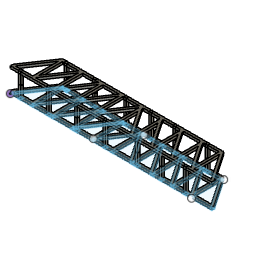
yamato (Autodesk Fusion 360 design; units mm, degrees)
Autodesk Fusion 360 part; units mm, degrees
note: some values were not read from the file. Chosen so that the rebuilt part matches the saved one: which bodies a step acts on; a direction.
sketch "Sketch1" plane through (0, 0, 0) normal (0, 0, 1) x (1, 0, 0)
  line L0 (0, 0) -> (250, 0)
  line L1 (250, 0) -> (250, 3)
  line L2 (250, 3) -> (0, 3)
  line L3 (0, 3) -> (0, 0)
  line L4 (25, 40) -> (225, 40)
  line L5 (225, 40) -> (225, 37)
  line L6 (225, 37) -> (25, 37)
  line L7 (25, 37) -> (25, 40)
  line L8 (225, 40) -> (250, 3)
  line L9 (250, 3) -> (247.5142, 1.3204)
  line L10 (247.5142, 1.3204) -> (222.5142, 38.3204)
  line L11 (222.5142, 38.3204) -> (225, 40)
  line L12 (25, 40) -> (0, 3)
  line L13 (0, 3) -> (2.4858, 1.3204)
  line L14 (2.4858, 1.3204) -> (27.4858, 38.3204)
  line L15 (27.4858, 38.3204) -> (25, 40)
  line L16 (50, 40) -> (53, 40)
  line L17 (53, 40) -> (53, 0)
  line L18 (53, 0) -> (50, 0)
  line L19 (50, 0) -> (50, 40)
  line L20 (75, 0) -> (75, 40)
  line L21 (78, 40) -> (78, 0)
  line L22 (75, 40) -> (78, 40)
  line L23 (78, 0) -> (75, 0)
  line L24 (100, 40) -> (103, 40)
  line L25 (100, 0) -> (100, 40)
  line L26 (103, 40) -> (103, 0)
  line L27 (103, 0) -> (100, 0)
  line L28 (128, 0) -> (125, 0)
  line L29 (125, 0) -> (125, 40)
  line L30 (128, 40) -> (128, 0)
  line L31 (125, 40) -> (128, 40)
  line L32 (150, 40) -> (153, 40)
  line L33 (150, 0) -> (150, 40)
  line L34 (153, 40) -> (153, 0)
  line L35 (153, 0) -> (150, 0)
  line L36 (178, 0) -> (175, 0)
  line L37 (175, 0) -> (175, 40)
  line L38 (178, 40) -> (178, 0)
  line L39 (175, 40) -> (178, 40)
  line L40 (200, 40) -> (203, 40)
  line L41 (200, 0) -> (200, 40)
  line L42 (203, 40) -> (203, 0)
  line L43 (203, 0) -> (200, 0)
  line L44 (225, 0) -> (225, 40)
  line L45 (25, 40) -> (28, 40)
  line L46 (25, 0) -> (25, 40)
  line L47 (28, 40) -> (28, 0)
  line L48 (28, 0) -> (25, 0)
  line L49 (222, 40) -> (225, 40)
  line L50 (222, 0) -> (222, 40)
  line L51 (225, 0) -> (222, 0)
  line L52 (197.5142, 38.3204) -> (200, 40)
  line L53 (200, 40) -> (225, 3)
  line L54 (222.5142, 1.3204) -> (197.5142, 38.3204)
  line L55 (225, 3) -> (222.5142, 1.3204)
  line L56 (172.5142, 38.3204) -> (175, 40)
  line L57 (175, 40) -> (200, 3)
  line L58 (197.5142, 1.3204) -> (172.5142, 38.3204)
  line L59 (200, 3) -> (197.5142, 1.3204)
  line L60 (147.5142, 38.3204) -> (150, 40)
  line L61 (150, 40) -> (175, 3)
  line L62 (172.5142, 1.3204) -> (147.5142, 38.3204)
  line L63 (175, 3) -> (172.5142, 1.3204)
  line L64 (122.5142, 38.3204) -> (125, 40)
  line L65 (125, 40) -> (150, 3)
  line L66 (147.5142, 1.3204) -> (122.5142, 38.3204)
  line L67 (150, 3) -> (147.5142, 1.3204)
  line L68 (25, 3) -> (27.4858, 1.3204)
  line L69 (27.4858, 1.3204) -> (52.4858, 38.3204)
  line L70 (50, 40) -> (25, 3)
  line L71 (52.4858, 38.3204) -> (50, 40)
  line L72 (50, 3) -> (52.4858, 1.3204)
  line L73 (52.4858, 1.3204) -> (77.4858, 38.3204)
  line L74 (75, 40) -> (50, 3)
  line L75 (77.4858, 38.3204) -> (75, 40)
  line L76 (75, 3) -> (77.4858, 1.3204)
  line L77 (77.4858, 1.3204) -> (102.4858, 38.3204)
  line L78 (100, 40) -> (75, 3)
  line L79 (102.4858, 38.3204) -> (100, 40)
  line L80 (0, 3) -> (2.4858, 1.3204)
  line L81 (2.4858, 1.3204) -> (27.4858, 38.3204)
  line L82 (25, 40) -> (0, 3)
  line L83 (27.4858, 38.3204) -> (25, 40)
  line L84 (100, 40) -> (75, 3)
  line L85 (75, 3) -> (77.4858, 1.3204)
  line L86 (77.4858, 1.3204) -> (102.4858, 38.3204)
  line L87 (102.4858, 38.3204) -> (100, 40)
  line L88 (127.4858, 38.3204) -> (125, 40)
  line L89 (125, 40) -> (100, 3)
  line L90 (102.4858, 1.3204) -> (127.4858, 38.3204)
  line L91 (100, 3) -> (102.4858, 1.3204)
  line L92 (30, 40) -> (33, 40)
  line L93 (33, 40) -> (33, 37)
  line L94 (33, 37) -> (30, 37)
  line L95 (30, 37) -> (30, 40)
  line L96 (65, 37) -> (65, 40)
  line L97 (65, 40) -> (68, 40)
  line L98 (68, 40) -> (68, 37)
  line L99 (68, 37) -> (65, 37)
  line L100 (30, 37) -> (30, 40)
  line L101 (30, 40) -> (33, 40)
  line L102 (33, 40) -> (33, 37)
  line L103 (33, 37) -> (30, 37)
  line L104 (104, 37) -> (104, 40)
  line L105 (104, 40) -> (107, 40)
  line L106 (107, 40) -> (107, 37)
  line L107 (107, 37) -> (104, 37)
  line L108 (135, 37) -> (135, 40)
  line L109 (135, 40) -> (138, 40)
  line L110 (138, 40) -> (138, 37)
  line L111 (138, 37) -> (135, 37)
  line L112 (165, 37) -> (165, 40)
  line L113 (165, 40) -> (168, 40)
  line L114 (168, 40) -> (168, 37)
  line L115 (168, 37) -> (165, 37)
  line L116 (205, 37) -> (205, 40)
  line L117 (205, 40) -> (208, 40)
  line L118 (208, 40) -> (208, 37)
  line L119 (208, 37) -> (205, 37)
  line L120 (30, 37) -> (30, 40)
  line L121 (30, 40) -> (33, 40)
  line L122 (33, 40) -> (33, 37)
  line L123 (33, 37) -> (30, 37)
  line L124 (10, 0) -> (10, 3)
  line L125 (10, 3) -> (13, 3)
  line L126 (13, 3) -> (13, 0)
  line L127 (13, 0) -> (10, 0)
  line L128 (45, 0) -> (45, 3)
  line L129 (45, 3) -> (48, 3)
  line L130 (48, 3) -> (48, 0)
  line L131 (48, 0) -> (45, 0)
  line L132 (80, 0) -> (80, 3)
  line L133 (80, 3) -> (83, 3)
  line L134 (83, 3) -> (83, 0)
  line L135 (83, 0) -> (80, 0)
  line L136 (115, 0) -> (115, 3)
  line L137 (115, 3) -> (118, 3)
  line L138 (118, 3) -> (118, 0)
  line L139 (118, 0) -> (115, 0)
  line L140 (155, 0) -> (155, 3)
  line L141 (155, 3) -> (158, 3)
  line L142 (158, 3) -> (158, 0)
  line L143 (158, 0) -> (155, 0)
  line L144 (185, 0) -> (185, 3)
  line L145 (185, 3) -> (188, 3)
  line L146 (188, 3) -> (188, 0)
  line L147 (188, 0) -> (185, 0)
  line L148 (215, 0) -> (215, 3)
  line L149 (215, 3) -> (218, 3)
  line L150 (218, 3) -> (218, 0)
  line L151 (218, 0) -> (215, 0)
  line L152 (30, 37) -> (30, 40)
  line L153 (30, 40) -> (33, 40)
  line L154 (33, 40) -> (33, 37)
  line L155 (33, 37) -> (30, 37)
  dimension "d1" = 250
  dimension "d2" = 3
  dimension "d3" = 200
  dimension "d4" = 3
  dimension "d5" = 3
  dimension "d7" = 3
  dimension "d8" = 3
  dimension "d9" = 3
  dimension "d10" = 3
  dimension "d11" = 3
  dimension "d12" = 3
  dimension "d13" = 3
  dimension "d14" = 3
  dimension "d16" = 3
  dimension "d17" = 3
  dimension "d18" = 3
  dimension "d19" = 3
  dimension "d20" = 3
  dimension "d21" = 3
  dimension "d22" = 3
  dimension "d23" = 3
  dimension "d24" = 3
  dimension "d25" = 3
  dimension "d26" = 3
  dimension "d27" = 3
  dimension "d32" = 3
  dimension "d33" = 3
  dimension "d34" = 3
  dimension "d35" = 3
  dimension "d36" = 3
  dimension "d37" = 3
  dimension "d38" = 3
  dimension "d39" = 3
  dimension "d40" = 3
  dimension "d41" = 3
  dimension "d42" = 3
  dimension "d43" = 3
  dimension "d44" = 3
  dimension "d45" = 3
  dimension "d46" = 3
  dimension "d47" = 3
  constraint coincident L0.start L3.end
  constraint perpendicular L8 L9
  constraint parallel L8 L10
  constraint parallel L9 L11
  constraint perpendicular L12 L13
  constraint parallel L12 L14
  constraint parallel L13 L15
  constraint perpendicular L16 L17
  constraint parallel L16 L18
  constraint parallel L17 L19
  constraint parallel L4 L16
  constraint coincident L4 L16.start
  constraint perpendicular L21 L22
  constraint parallel L22 L23
  constraint parallel L20 L21
  constraint perpendicular L24 L26
  constraint parallel L24 L27
  constraint parallel L25 L26
  constraint perpendicular L30 L31
  constraint parallel L28 L31
  constraint parallel L29 L30
  constraint perpendicular L32 L34
  constraint parallel L32 L35
  constraint parallel L33 L34
  constraint perpendicular L38 L39
  constraint parallel L36 L39
  constraint parallel L37 L38
  constraint perpendicular L40 L42
  constraint parallel L40 L43
  constraint parallel L41 L42
  constraint perpendicular L45 L47
  constraint parallel L45 L48
  constraint parallel L46 L47
  constraint parallel L49 L51
  constraint perpendicular L53 L55
  constraint parallel L53 L54
  constraint parallel L52 L55
  constraint perpendicular L57 L59
  constraint parallel L57 L58
  constraint parallel L56 L59
  constraint perpendicular L61 L63
  constraint parallel L61 L62
  constraint parallel L60 L63
  constraint perpendicular L65 L67
  constraint parallel L65 L66
  constraint parallel L64 L67
  constraint perpendicular L68 L70
  constraint parallel L69 L70
  constraint parallel L68 L71
  constraint perpendicular L72 L74
  constraint parallel L73 L74
  constraint parallel L72 L75
  constraint perpendicular L76 L78
  constraint parallel L77 L78
  constraint parallel L76 L79
  constraint perpendicular L80 L82
  constraint parallel L81 L82
  constraint parallel L80 L83
  constraint perpendicular L84 L85
  constraint parallel L84 L86
  constraint parallel L85 L87
  constraint horizontal L92
  constraint vertical L93
  constraint horizontal L94
  constraint vertical L95
  constraint coincident L4 L92.start
  constraint horizontal L97
  constraint vertical L98
  constraint horizontal L99
  constraint vertical L96
  constraint horizontal L101
  constraint vertical L102
  constraint horizontal L103
  constraint vertical L100
  constraint horizontal L105
  constraint vertical L106
  constraint horizontal L107
  constraint vertical L104
  constraint horizontal L109
  constraint vertical L110
  constraint horizontal L111
  constraint vertical L108
  constraint horizontal L113
  constraint vertical L114
  constraint horizontal L115
  constraint vertical L112
  constraint horizontal L117
  constraint vertical L118
  constraint horizontal L119
  constraint vertical L116
  constraint horizontal L121
  constraint vertical L122
  constraint horizontal L123
  constraint vertical L120
  constraint horizontal L125
  constraint vertical L126
  constraint horizontal L127
  constraint vertical L124
  constraint horizontal L129
  constraint vertical L130
  constraint horizontal L131
  constraint vertical L128
  constraint horizontal L133
  constraint vertical L134
  constraint horizontal L135
  constraint vertical L132
  constraint horizontal L137
  constraint vertical L138
  constraint horizontal L139
  constraint vertical L136
  constraint horizontal L141
  constraint vertical L142
  constraint horizontal L143
  constraint vertical L140
  constraint horizontal L145
  constraint vertical L146
  constraint horizontal L147
  constraint vertical L144
  constraint horizontal L149
  constraint vertical L150
  constraint horizontal L151
  constraint vertical L148
  constraint horizontal L153
  constraint vertical L154
  constraint horizontal L155
  constraint vertical L152
  measures "d1" distance of L0.start L0.end
  measures "d2" distance of L0.start L2.end
  measures "d3" distance of L4.start L4.end
  measures "d4" distance of L4.start L6.end
  measures "d5" distance of L4.end L10.end
  measures "d7" distance of L4.start L14.end
  measures "d8" distance of L16.start L16.end
  measures "d9" distance of L21.start L20.end
  measures "d10" distance of L24.end L24.start
  measures "d11" distance of L29.end L30.start
  measures "d12" distance of L32.end L32.start
  measures "d13" distance of L37.end L38.start
  measures "d14" distance of L40.end L40.start
  measures "d16" distance of L45.end L4.start
  measures "d17" distance of L49.start L4.end
  measures "d18" distance of L52.start L40.start
  measures "d19" distance of L56.start L37.end
  measures "d20" distance of L60.start L32.start
  measures "d21" distance of L64.start L29.end
  measures "d22" distance of L16.start L69.end
  measures "d23" distance of L20.end L73.end
  measures "d24" distance of L24.start L77.end
  measures "d25" distance of L4.start L14.end
  measures "d26" distance of L24.start L77.end
  measures "d27" distance of L29.end L88.start
  measures "d32" distance of L92.start L92.end
  measures "d33" distance of L96.end L97.end
  measures "d34" distance of L92.start L92.end
  measures "d35" distance of L104.end L105.end
  measures "d36" distance of L108.end L109.end
  measures "d37" distance of L112.end L113.end
  measures "d38" distance of L116.end L117.end
  measures "d39" distance of L92.start L92.end
  measures "d40" distance of L124.end L125.end
  measures "d41" distance of L128.end L129.end
  measures "d42" distance of L132.end L133.end
  measures "d43" distance of L136.end L137.end
  measures "d44" distance of L140.end L141.end
  measures "d45" distance of L144.end L145.end
  measures "d46" distance of L148.end L149.end
  measures "d47" distance of L92.start L92.end
extrude "Extrude2" add sketch "Sketch1" along normal blind 15 contours L0 L2 L124 L125 L126 L127 | L4 L6 L92 L93 L94 L95 L100 L101 L102 L103 L120 L121 L122 L123 L152 L153 L154 L155 | L0 L2 L128 L129 L130 L131 | L4 L6 L96 L97 L98 L99 | L0 L2 L132 L133 L134 L135 | L4 L6 L104 L105 L106 L107 | L0 L2 L136 L137 L138 L139 | L4 L6 L108 L109 L110 L111 | L0 L2 L140 L141 L142 L143 | L4 L6 L112 L113 L114 L115 | L4 L6 L116 L117 L118 L119 | L0 L2 L148 L149 L150 L151 makes body 1 at (166, 40, 5) makes body 2 at (117, 3, 5) makes body 3 at (66, 40, 5) makes body 4 at (12, 3, 5) makes body 5 at (106, 37, 5) makes body 6 at (206, 40, 5) makes body 7 at (157, 3, 5) makes body 8 at (82, 3, 5) makes body 9 at (31, 40, 5) makes body 10 at (47, 3, 5) makes body 11 at (136, 40, 5) makes body 12 at (217, 3, 5)
extrude "Extrude1" add sketch "Sketch1" along normal blind 3 separate body contours L0 L2 L3 L13 L14 L80 L81 L124 | L0 L2 L124 L125 L126 L127 | L2 L7 L12 L14 L46 L81 L82 | L2 L13 L14 L80 L81 | L0 L2 L46 L126 | L6 L7 L14 L15 L46 L81 L83 | L4 L6 L14 L15 L45 L47 L81 L83 | L0 L46 L47 L48 L68 L69 | L6 L14 L46 L81 | L6 L14 L46 L47 L70 L81 | L4 L6 L47 L95 L100 L120 L152 | L0 L2 L47 L69 L128 | L2 L47 L70 | L2 L47 L68 L69 | L4 L6 L92 L93 L94 L95 L100 L101 L102 L103 L120 L121 L122 L123 L152 L153 L154 L155 | L0 L2 L128 L129 L130 L131 | L2 L47 L69 | L2 L6 L19 L47 L69 L70 | L4 L6 L70 L93 L102 L122 L154 | L0 L2 L19 L130 | L6 L19 L70 | L6 L19 L69 L71 | L4 L6 L16 L17 L69 L71 | L0 L17 L18 L19 L72 L73 | L6 L17 L19 L69 L74 | L6 L19 L69 | L4 L6 L17 L96 | L0 L2 L17 L20 L73 | L2 L17 L74 | L2 L17 L72 L73 | L4 L6 L96 L97 L98 L99 | L0 L20 L21 L23 L76 L77 L85 L86 | L2 L17 L73 | L2 L6 L17 L20 L73 L74 | L4 L6 L74 L98 | L0 L2 L21 L77 L86 L132 | L2 L21 L78 L84 | L2 L21 L76 L77 L85 L86 | L6 L20 L21 L73 L78 L84 | L6 L20 L74 | L6 L20 L73 L75 | L4 L6 L21 L22 L73 L75 | L0 L2 L132 L133 L134 L135 | L2 L21 L77 L86 | L2 L6 L21 L25 L77 L78 L84 L86 | L6 L20 L73 | L4 L6 L21 L78 L84 | L0 L2 L25 L134 | L6 L25 L78 L84 | L6 L25 L77 L79 L86 L87 | L4 L6 L24 L26 L77 L79 L86 L87 | L0 L25 L26 L27 L90 L91 | L6 L25 L26 L77 L86 L89 | L6 L25 L77 L86 | L4 L6 L26 L104 | L0 L2 L26 L90 L136 | L2 L26 L89 | L2 L26 L90 L91 | L4 L6 L104 L105 L106 L107 | L0 L2 L136 L137 L138 L139 | L2 L26 L90 | L2 L6 L26 L66 L89 L90 | L4 L6 L64 L66 L89 L106 | L0 L2 L29 L138 | L6 L66 L89 | L6 L29 L65 L90 | L64 L66 L89 | L65 L88 L90 | L4 L6 L30 L31 L65 L88 L90 | L6 L29 L66 L89 | L0 L2 L28 L29 L30 | L2 L29 L30 L66 | L6 L29 L66 | L6 L30 L65 L66 L90 | L6 L29 L90 | L4 L6 L30 L108 | L6 L65 L90 | L0 L2 L30 L33 L66 L67 | L2 L30 L65 L66 | L4 L6 L108 L109 L110 L111 | L6 L30 L65 | L0 L2 L33 L34 L35 | L2 L66 L67 | L4 L6 L60 L62 L110 | L0 L2 L34 L140 | L2 L33 L34 L62 | L6 L33 L61 | L6 L33 L60 L62 | L4 L6 L32 L34 L61 | L0 L2 L140 L141 L142 L143 | L6 L33 L62 | L6 L33 L34 L61 L62 | L4 L6 L34 L112 | L6 L34 L61 | L0 L2 L37 L62 L63 L142 | L2 L34 L61 L62 | L4 L6 L112 L113 L114 L115 | L0 L2 L36 L37 L38 | L2 L62 L63 | L4 L6 L56 L58 L114 | L2 L37 L38 L58 | L0 L2 L38 L144 | L6 L37 L57 | L6 L37 L56 L58 | L4 L6 L38 L39 L57 | L6 L37 L58 | L6 L37 L38 L57 L58 | L0 L2 L144 L145 L146 L147 | L4 L6 L38 L52 L54 | L6 L38 L57 | L2 L38 L57 L58 | L0 L2 L41 L58 L59 L146 | L6 L41 L53 | L6 L41 L52 L54 | L4 L6 L40 L42 L53 | L2 L58 L59 | L0 L2 L41 L42 L43 | L4 L6 L42 L116 | L6 L41 L54 | L6 L41 L42 L53 L54 | L6 L42 L53 | L2 L41 L42 L54 | L0 L2 L42 L148 | L4 L6 L116 L117 L118 L119 | L2 L42 L50 L53 L54 | L0 L2 L148 L149 L150 L151 | L4 L6 L50 L118 | L2 L50 L53 | L6 L10 L44 L50 L53 | L0 L2 L50 L54 L150 | L4 L6 L10 L11 L49 L50 | L2 L50 L54 | L2 L50 L54 L55 | L0 L1 L2 L9 L10 L44 | L0 L44 L50 L51 L54 L55 | L2 L5 L8 L10 L44 | L5 L6 L10 L11 L44 | L6 L10 L44 | L2 L9 L10 makes body 13
extrude "Extrude3" cut sketch "Sketch1" along normal blind 41 contours L0 L2 L144 L145 L146 L147 bodies 13
extrude "Extrude4" add sketch "Sketch1" along normal blind 15 contours L0 L2 L144 L145 L146 L147 bodies 13
ref_plane "WorkPlane1" through (105.5, 38.5, 15) normal (0, 0, 1) x (1, 0, 0)
mirror "Mirror1" about plane through (105.5, 38.5, 15) normal (0, 0, 1) of bodies 1 6 7 5 12 9 3 10 4 8 11 2 13 makes body 14 at (132.1265, 1, 30) makes body 15 at (166, 40, 25) makes body 16 at (117, 3, 25) makes body 17 at (66, 40, 25) makes body 18 at (12, 3, 25) makes body 19 at (106, 37, 25) makes body 20 at (206, 40, 25) makes body 21 at (157, 3, 25) makes body 22 at (82, 3, 25) makes body 23 at (31, 40, 25) makes body 24 at (47, 3, 25) makes body 25 at (136, 40, 25) makes body 26 at (217, 3, 25)
